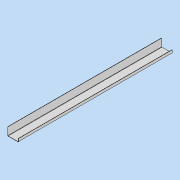
# Autodesk Inventor part: Dragchian_Holder
Saved by Autodesk Inventor 2020 (Build 240168000, 168)
## iProperties
Created: 2021-07-13
Part Number: Dragchian_Holder
Material: 一般
Document SubType Name: Sheet Metal
Designer: magnarecta
Density: 1 g/cm^3
Sheet Metal Rule: Default_mm
Appearance: 既定
Author: magnarecta
Autodesk Inventor part; units mm, degrees
ref_plane "YZ Plane" through (0, 0, 0) normal (1, 0, 0) x (0, 1, 0)
ref_plane "XZ Plane" through (0, 0, 0) normal (0, 1, 0) x (-1, 0, 0)
ref_plane "XY Plane" through (0, 0, 0) normal (0, 0, 1) x (1, 0, 0)
sketch "スケッチ1" plane through (0, 0, 0) normal (1, 0, 0) x (0, 1, 0)
  line L0 (0, 0) -> (52, 0)
  line L1 (52, 0) -> (52, 1000)
  line L2 (52, 1000) -> (0, 1000)
  line L3 (0, 1000) -> (0, 0)
  dimension "d0" = 52
  dimension "d1" = 1000
  measures "d0" distance of L0.start L0.end
  measures "d1" distance of L2.end L0.start
extrude "プレート1" add sketch "スケッチ1" along normal blind 1.5
sketch "スケッチ2" plane through (0, 1.5, 0) normal (0, -1, 0) x (1, 0, 0)
  line L0 (0, 1000) -> (0, 0)
  line L1 (0, 0) -> (70, 0)
  line L2 (70, 0) -> (70, 1000)
  line L3 (70, 1000) -> (0, 1000)
  constraints: 6 end point, 1 horizontal, 1 perpendicular, 1 vertical
edge flange "フランジ1" height 70 angle 90 thickness 1.5 bend radius 1.5 thickness toward (0, -1, 0) relief straight relief width 1.5 relief depth 0.75 edges at (1.5, 0, 500) wall of the first edge with corners at (0, 1.5, 1000) (0, 1.5, 0) (70, 1.5, 0) (70, 1.5, 1000)
bend "曲げ1"
corner "コーナー1"
sketch "スケッチ3" plane through (68.5, 0, 0) normal (1, 0, 0) x (0, 1, 0)
  line L0 (0, 1000) -> (0, 0)
  line L1 (0, 0) -> (20, 0)
  line L2 (20, 0) -> (20, 1000)
  line L3 (20, 1000) -> (0, 1000)
  constraints: 6 end point, 1 horizontal, 1 perpendicular, 1 vertical
edge flange "フランジ2" height 20 angle 90 thickness 1.5 bend radius 1.5 thickness toward (1, 0, 0) relief straight relief width 1.5 relief depth 0.75 edges at (70, 1.5, 500) wall of the first edge with corners at (68.5, 0, 1000) (68.5, 0, 0) (68.5, 20, 0) (68.5, 20, 1000)
bend "曲げ2"
corner "コーナー2"
fillet "フィレット1" radius 2 4 edges at (0.75, 52, 1000) (69.25, 20, 1000) (0.75, 52, 0) (69.25, 20, 0)
equation "\"d2\" = Thickness"
equation "\"d3\" = BendReliefWidth"
equation "\"d4\" = BendReliefDepth"
equation "\"d5\" = MinimumRemnant"
equation "\"d6\" = TransitionRadius"
equation "\"d9\" = BendRadius"
equation "\"d10\" = CornerReliefSize"
equation "\"d11\" = GapSize"
equation "\"d12\" = JacobiRadiusSize"
equation "\"d13\" = BendReliefWidth"
equation "\"d14\" = BendReliefDepth"
equation "\"d15\" = MinimumRemnant"
equation "\"d16\" = TransitionRadius"
equation "\"d19\" = BendRadius"
equation "\"d20\" = CornerReliefSize"
equation "\"d21\" = GapSize"
equation "\"d22\" = JacobiRadiusSize"
equation "\"BendRadius\" = Thickness"
equation "\"BendReliefWidth\" = Thickness"
equation "\"BendReliefDepth\" = 0.5 * Thickness"
equation "\"CornerReliefSize\" = 4 * Thickness"
equation "\"MinimumRemnant\" = 2 * Thickness"
equation "\"TransitionRadius\" = BendRadius"
equation "\"JacobiRadiusSize\" = BendRadius"
equation "\"GapSize\" = Thickness"
equation "\"Thickness\" = 1.5"
